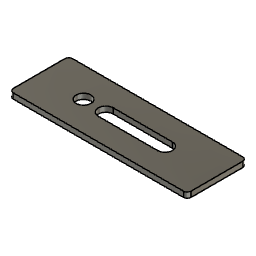
Chain Guard Bracket v1 (Autodesk Fusion 360 design; units mm, degrees)
Autodesk Fusion 360 part; units mm, degrees
sketch "Sketch1" plane through (0, 0, 0) normal (0, 0, 1) x (1, 0, 0) in component "Chain Guard"
  line L0 (0, 0) -> (76.2, 0)
  line L1 (76.2, 0) -> (76.2, 25.4)
  line L2 (76.2, 25.4) -> (0, 25.4)
  line L3 (0, 25.4) -> (0, 0)
  line L4 (0, 12.7) -> (76.2, 12.7) construction
  circle A0 centre (19.05, 12.7) radius 3.175
  line L5 (28.575, 9.525) -> (53.975, 9.525)
  arc A1 (53.975, 9.525) -> (53.975, 15.875) centre (53.975, 12.7) ccw
  line L6 (53.975, 15.875) -> (28.575, 15.875)
  arc A2 (28.575, 15.875) -> (28.575, 9.525) centre (28.575, 12.7) ccw
  line L7 (28.575, 12.7) -> (53.975, 12.7) construction
  dimension "d2" = 76.2
  dimension "d3" = 25.4
  dimension "d4" = 6.35
  dimension "d5" = 19.05
  dimension "d6" = 6.35
  dimension "d7" = 28.575
  dimension "d8" = 25.4
  constraint horizontal L0
  constraint vertical L1
  constraint horizontal L2
  constraint vertical L3
  constraint coincident L0.start L3.end
  constraint midpoint L3 L4.start
  constraint midpoint L1 L4.end
  constraint coincident L4 A0.centre
  constraint tangent L5 A1
  constraint tangent A1 L6
  constraint parallel L5 L6
  constraint tangent L6 A2
  constraint tangent L5 A2
  constraint coincident L4 A1.centre
  constraint perpendicular L3 L7
  measures "d2" distance of L0.start L0.end
  measures "d3" distance of L0.start L2.end
  measures "d4" diameter of A0
  measures "d5" distance of L4.start A0.centre
  measures "d6" distance of L5 L6
  measures "d7" horizontal distance of L2.end A2.centre
  measures "d8" distance of A2.centre A1.centre
extrude "Extrude1" add sketch "Sketch1" along normal blind 2.3114 in component "Chain Guard"
fillet "Fillet1" radius 1.5875 4 edges at (76.2, 0, 1.1557) (76.2, 25.4, 1.1557) (0, 25.4, 1.1557) (0, 0, 1.1557) in component "Chain Guard"
component "Chain Guard" placed x (1, 0, 0) y (0, 1, 0) z (0, 0, 1) at (0, 0, 0)
